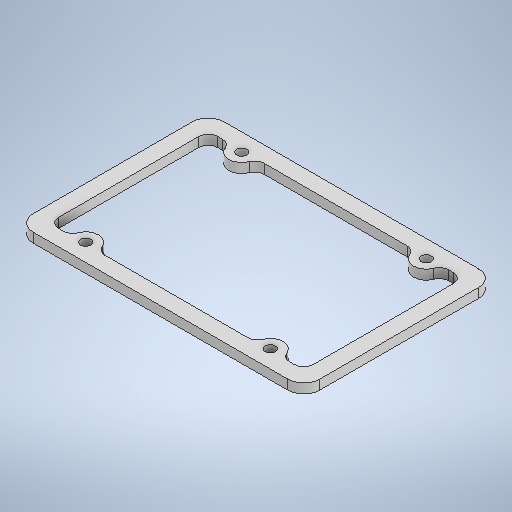
# Autodesk Inventor part: RemoteDisplayMount
Saved by Autodesk Inventor 2025 (Build 290162000, 162)
## iProperties
Created: 2025-05-02
Part Number: RemoteDisplayMount
Material: Generic
Document SubType Name: Modeling
Designer: tvoko
Density: 1 g/cm^3
Appearance: Default
Author: tvoko
Autodesk Inventor part; units mm, degrees
ref_plane "YZ Plane" through (0, 0, 0) normal (1, 0, 0) x (0, 1, 0)
ref_plane "XZ Plane" through (0, 0, 0) normal (0, 1, 0) x (-1, 0, 0)
ref_plane "XY Plane" through (0, 0, 0) normal (0, 0, 1) x (1, 0, 0)
sketch "Sketch1" plane through (0, 0, 0) normal (0, 1, 0) x (-1, 0, 0)
  line L0 (0, 0) -> (58, 0) construction
  line L1 (58, 0) -> (58, -49) construction
  line L2 (58, -49) -> (0, -49) construction
  line L3 (0, -49) -> (0, 0) construction
  circle A0 centre (58, -49) radius 1.6
  circle A1 centre (0, -49) radius 1.6
  circle A2 centre (58, 0) radius 1.6
  circle A3 centre (0, 0) radius 1.6
  line L4 (74, -24.5) -> (-16, -24.5) construction
  line L5 (29, -54.5) -> (29, 5.5) construction
  line L6 (69, -54.5) -> (-11, -54.5)
  line L7 (-16, -49.5) -> (-16, 0.5)
  line L8 (-11, 5.5) -> (69, 5.5)
  line L9 (74, 0.5) -> (74, -49.5)
  arc A4 (69, -54.5) -> (74, -49.5) centre (69, -49.5) ccw
  arc A5 (-16, -49.5) -> (-11, -54.5) centre (-11, -49.5) ccw
  arc A6 (-11, 5.5) -> (-16, 0.5) centre (-11, 0.5) ccw
  arc A7 (74, 0.5) -> (69, 5.5) centre (69, 0.5) ccw
  line L10 (-8, -49.5) -> (-6.5383, -49.5)
  line L11 (69, -46.5) -> (69, -2.5)
  line L12 (66, 0.5) -> (64.5383, 0.5)
  line L13 (-11, -2.5) -> (-11, -46.5)
  arc A8 (61.7362, -47.5714) -> (54.2638, -47.5714) centre (58, -49) ccw
  arc A9 (3.7362, -47.5714) -> (-3.7362, -47.5714) centre (0, -49) ccw
  arc A10 (-3.7362, -1.4286) -> (3.7362, -1.4286) centre (0, 0) ccw
  arc A11 (54.2638, -1.4286) -> (61.7362, -1.4286) centre (58, 0) ccw
  arc A12 (54.0314, -49.5) -> (61.9686, -49.5) centre (58, -49) ccw construction
  arc A13 (-3.9686, -49.5) -> (3.9686, -49.5) centre (0, -49) ccw construction
  arc A14 (3.9686, 0.5) -> (-3.9686, 0.5) centre (0, 0) ccw construction
  arc A15 (61.9686, 0.5) -> (54.0314, 0.5) centre (58, 0) ccw construction
  line L14 (64.5383, -49.5) -> (66, -49.5)
  line L15 (51.4617, 0.5) -> (6.5383, 0.5)
  line L16 (-6.5383, 0.5) -> (-8, 0.5)
  line L17 (6.5383, -49.5) -> (51.4617, -49.5)
  arc A16 (61.7362, -47.5714) -> (64.5383, -49.5) centre (64.5383, -46.5) ccw
  arc A17 (51.4617, -49.5) -> (54.2638, -47.5714) centre (51.4617, -46.5) ccw
  arc A18 (64.5383, 0.5) -> (61.7362, -1.4286) centre (64.5383, -2.5) ccw
  arc A19 (54.2638, -1.4286) -> (51.4617, 0.5) centre (51.4617, -2.5) ccw
  arc A20 (6.5383, 0.5) -> (3.7362, -1.4286) centre (6.5383, -2.5) ccw
  arc A21 (-3.7362, -1.4286) -> (-6.5383, 0.5) centre (-6.5383, -2.5) ccw
  arc A22 (-6.5383, -49.5) -> (-3.7362, -47.5714) centre (-6.5383, -46.5) ccw
  arc A23 (3.7362, -47.5714) -> (6.5383, -49.5) centre (6.5383, -46.5) ccw
  arc A24 (66, -49.5) -> (69, -46.5) centre (66, -46.5) ccw
  arc A25 (69, -2.5) -> (66, 0.5) centre (66, -2.5) ccw
  arc A26 (-8, 0.5) -> (-11, -2.5) centre (-8, -2.5) ccw
  arc A27 (-11, -46.5) -> (-8, -49.5) centre (-8, -46.5) ccw
  point P0 (29, -49)
  point P1 (0, -24.5)
  point P2 (58, -24.5)
  point P3 (29, 0)
  point P4 (29, -24.5)
  dimension "d0" = 3.2
  dimension "d1" = 58
  dimension "d2" = 49
  dimension "d3" = 5
  dimension "d4" = 90
  dimension "d5" = 60
  dimension "d6" = 5
  dimension "d7" = 8
  dimension "d8" = 5
  dimension "d9" = 5
  dimension "d10" = 5
  dimension "d11" = 3
  constraints: 56 point on circle, 36 end point, 32 tangent, 28 centre point, 20 equal radius, 20 point on line, 14 parallel, 10 midpoint, 8 coincident, 5 perpendicular, 2 horizontal
  measures "d0" diameter of A0
  measures "d1" distance of L1.end L2.end
  measures "d2" distance of L2.end L0.start
  measures "d3" radius of A4
  measures "d4" distance of L4.start L4.end
  measures "d5" distance between parallel lines of L8 L6
  measures "d6" distance between parallel lines of L6 L10
  measures "d7" diameter of A8
  measures "d8" distance between parallel lines of L9 L11
  measures "d9" distance between parallel lines of L7 L13
  measures "d10" distance between parallel lines of L8 L15
  measures "d11" radius of A16
extrude "Extrusion1" add sketch "Sketch1" along normal blind 3
equation "\"d8\" = d6"
equation "\"d9\" = d6"
equation "\"d10\" = d6"
body "Solid1"
